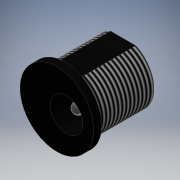
# Autodesk Inventor part: Barrel_Jack
Saved by Autodesk Inventor 2016 (Build 200138000, 138)
## iProperties
Created: 2016-05-21
Part Number: Barrel_Jack
Material: PC/ABS Plastic
Document SubType Name: Modeling
Designer: agmle
Density: 0.357273 g/cm^3
Appearance: Smooth - Black
Mass: 0.385283 g
Surface Area: 9.70299 cm^2
Volume: 1.0784 cm^3
Barrel_OD: 11.500 mm
Barrel_Flat_Width: 10.500 mm
Author: agmle
Autodesk Inventor part; units mm, degrees
ref_plane "YZ Plane" through (0, 0, 0) normal (1, 0, 0) x (0, 1, 0)
ref_plane "XZ Plane" through (0, 0, 0) normal (0, 1, 0) x (-1, 0, 0)
ref_plane "XY Plane" through (0, 0, 0) normal (0, 0, 1) x (1, 0, 0)
sketch "Sketch1" plane through (0, 0, 0) normal (0, 1, 0) x (-1, 0, 0)
  circle A0 centre (0, 0) radius 6.86
  dimension "d0" = 13.72
  constraints: 1 centre point, 1 coincident
  measures "d0" diameter of A0
extrude "Extrusion1" add sketch "Sketch1" along normal blind 1.5
sketch "Sketch2" plane through (0, 1.5, 0) normal (0, 1, 0) x (1, 0, 0)
  line L0 (-2.3452, -5.25) -> (2.3452, -5.25)
  line L1 (2.3452, 5.25) -> (-2.3452, 5.25)
  line L2 (0, 0) -> (0, 5.25) construction
  line L3 (0, 0) -> (0, -5.25) construction
  arc A0 (2.3452, -5.25) -> (2.3452, 5.25) centre (0, 0) ccw
  arc A1 (-2.3452, 5.25) -> (-2.3452, -5.25) centre (0, 0) ccw
  dimension "Barrel_Flat_Width" = 10.5
  dimension "d5" = 5.75
  constraints: 8 end point, 4 point on circle, 2 centre point, 2 collinear, 2 midpoint, 1 coincident, 1 concentric, 1 horizontal, 1 parallel
  measures "Barrel_Flat_Width" distance between parallel lines of L1 L0
  measures "d5" radius of A1
extrude "Extrusion2" add sketch "Sketch2" along normal blind 10.86
thread "Thread1" size "M12x0.75" class "6g" standard "ANSI Metric M Profile" full length
thread "Thread2" size "M12x0.75" class "6g" standard "ANSI Metric M Profile" full length
sketch "Sketch3" plane through (0, 0, 0) normal (0, -1, 0) x (1, 0, 0)
  circle A0 centre (1.81, 0) radius 3.05
  line L0 (0, 0) -> (1.81, 0) construction
  circle A1 centre (0, 0) radius 6.86 construction
  dimension "d12" = 6.1
  dimension "d14" = 2
  constraints: 2 end point, 1 centre point, 1 horizontal
  measures "d12" diameter of A0
extrude "Extrusion3" cut sketch "Sketch3" against normal blind 9
sketch "Sketch4" plane through (1.81, 9, 0) normal (0, -1, 0) x (1, 0, 0)
  circle A0 centre (0, 0) radius 3.05 construction
  circle A1 centre (0, 0) radius 1.05
  point P0 (-1.81, 0)
  dimension "d17" = 2.1
  constraints: 1 centre point, 1 coincident
  measures "d17" diameter of A1
extrude "Extrusion4" add sketch "Sketch4" along normal blind 7.83
fillet "Fillet1" radius 1.05 1 edges at (0.76, 1.17, 0)
body "Solid1"
